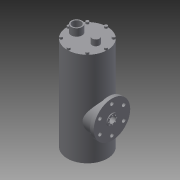
# Autodesk Inventor part: x-ray tube
Saved by Autodesk Inventor 2015 (Build 190159000, 159)
## iProperties
Created: 2014-11-30
Part Number: x-ray tube
Material: Generic
Document SubType Name: Modeling
Designer: Andrew
Density: 1 g/cm^3
Appearance: Default
Author: Andrew
Autodesk Inventor part; units mm, degrees
ref_plane "YZ Plane" through (0, 0, 0) normal (1, 0, 0) x (0, 1, 0)
ref_plane "XZ Plane" through (0, 0, 0) normal (0, 1, 0) x (-1, 0, 0)
ref_plane "XY Plane" through (0, 0, 0) normal (0, 0, 1) x (1, 0, 0)
sketch "Sketch1" plane through (0, 0, 0) normal (0, 1, 0) x (-1, 0, 0)
  circle A0 centre (0, 0) radius 34.925
  dimension "d0" = 69.85
  constraints: 1 centre point, 1 coincident
  measures "d0" diameter of A0
extrude "Extrusion1" add sketch "Sketch1" along normal blind 163.576
sketch "Sketch2" plane through (0, 0, 0) normal (1, 0, 0) x (0, 1, 0)
  circle A0 centre (62.738, 0) radius 28.575
  line L0 (0, 34.925) -> (0, -34.925) projected
  line L1 (163.576, -34.925) -> (163.576, 34.925) projected
  point P0 (0, 0)
  dimension "d3" = 100.838
  dimension "d4" = 57.15
  constraints: 1 centre point
  measures "d3" distance from line of A0.centre L1
  measures "d4" diameter of A0
extrude "Extrusion2" add sketch "Sketch2" along normal blind 36.449
sketch "Sketch3" plane through (36.449, 62.738, 0) normal (1, 0, 0) x (0, 0, -1)
  circle A0 centre (0, 0) radius 31.75
  point P0 (0, -62.738)
  dimension "d7" = 63.5
  constraints: 1 centre point
  measures "d7" diameter of A0
extrude "Extrusion3" add sketch "Sketch3" along normal blind 6.35
sketch "Sketch4" plane through (36.449, 62.738, 0) normal (-1, 0, 0) x (0, 0, 1)
  circle A0 centre (0, 0) radius 29.21
  point P0 (0, -62.738)
  dimension "d10" = 58.42
  constraints: 1 centre point
  measures "d10" diameter of A0
extrude "Extrusion4" add sketch "Sketch4" along normal blind 1.4859
sketch "Sketch5" plane through (42.799, 62.738, 0) normal (1, 0, 0) x (0, 0, -1)
  circle A0 centre (0, 0) radius 31.75 construction
  circle A1 centre (0, 0) radius 23.8125 construction
  circle A2 centre (0, 23.8125) radius 3.175
  line L0 (0, -95.4532) -> (0, 133.5532) construction
  circle A3 centre (-20.6222, 11.9063) radius 3.175
  circle A4 centre (-20.6222, -11.9062) radius 3.175
  circle A5 centre (0, -23.8125) radius 3.175
  circle A6 centre (20.6222, -11.9063) radius 3.175
  circle A7 centre (20.6222, 11.9062) radius 3.175
  circle A8 centre (0, 0) radius 5.715
  circle A9 centre (0, 0) radius 31.75 projected
  circle A10 centre (0, 0) radius 9.525
  circle A11 centre (0, 6.985) radius 0.9525
  circle A12 centre (-4.9391, 4.9391) radius 0.9525
  circle A13 centre (-6.985, 0) radius 0.9525
  circle A14 centre (-4.9391, -4.9391) radius 0.9525
  circle A15 centre (0, -6.985) radius 0.9525
  circle A16 centre (4.9391, -4.9391) radius 0.9525
  circle A17 centre (6.985, 0) radius 0.9525
  circle A18 centre (4.9391, 4.9391) radius 0.9525
  point P0 (0, -62.738)
  dimension "d13" = 47.625
  dimension "d14" = 6.35
  dimension "d17" = 360
  dimension "d19" = 11.43
  dimension "d20" = 19.05
  dimension "d21" = 1.905
  dimension "d22" = 6.985
  dimension "d25" = 360
  constraints: 16 centre point, 3 coincident, 2 point on line, 1 vertical alignment, 32 other
  measures "d14" diameter of A2
  measures "d19" diameter of A8
  measures "d20" diameter of A10
  measures "d21" diameter of A11
  measures "d22" distance of A0.centre A11.centre
extrude "Extrusion5" cut sketch "Sketch5" against normal blind 5.715 contours A2 | A3 | A4 | A5 | A6 | A7
extrude "Extrusion6" cut sketch "Sketch5" against normal blind 5.715 contours A11 | A12 | A13 | A14 | A15 | A16 | A17 | A18
extrude "Extrusion7" cut sketch "Sketch5" against normal blind 50.8 contours A8
extrude "Extrusion8" add sketch "Sketch5" along normal blind 1.27 contours A10
sketch "Sketch6" plane through (0, 163.576, 0) normal (0, 1, 0) x (1, 0, 0)
  circle A0 centre (0, 0) radius 34.925 projected
  circle A1 centre (14.6864, 0) radius 6.35
  circle A2 centre (-18.669, 0) radius 9.525
  circle A3 centre (0, -32.385) radius 2.54
  line L0 (0, 48.895) -> (0, -48.895) projected
  line L1 (59.8678, 0) -> (-50.7238, 0) projected
  circle A4 centre (0, 0) radius 29.845
  circle A5 centre (22.8997, -22.8997) radius 2.54
  circle A6 centre (32.385, 0) radius 2.54
  circle A7 centre (22.8997, 22.8997) radius 2.54
  circle A8 centre (0, 32.385) radius 2.54
  circle A9 centre (-22.8997, 22.8997) radius 2.54
  circle A10 centre (-32.385, 0) radius 2.54
  circle A11 centre (-22.8997, -22.8997) radius 2.54
  line L2 (-34.925, -31.1615) -> (-34.925, 23.8469) construction
  circle A12 centre (-18.669, 0) radius 7.62
  dimension "d35" = 5.08
  dimension "d38" = 360
  dimension "d40" = 16.256
  dimension "d41" = 12.7
  dimension "d42" = 19.05
  dimension "d43" = 15.24
  constraints: 12 centre point, 3 point on line, 3 tangent, 2 end point, 1 coincident, 1 parallel, 1 vertical, 17 other
  measures "d35" diameter of A3
  measures "d40" distance from line of L2 A2.centre
  measures "d41" diameter of A1
  measures "d42" diameter of A2
  measures "d43" diameter of A12
extrude "Extrusion9" add sketch "Sketch6" along normal blind 3.175 contours A6 L1 | L1 A6 | A7 | A5 | A8 L0 | L0 A8 | L0 A3 | A3 L0 | A9 | A11 | A10 L1 | L1 A10
extrude "Extrusion10" cut sketch "Sketch6" against normal blind 50.8 contours A12 L1 | L1 A12
extrude "Extrusion11" add sketch "Sketch6" along normal blind 12.7 contours L1 A12 A2 | A2 L1 A12
extrude "Extrusion12" add sketch "Sketch6" along normal blind 10.16 contours L1 A1 | A1 L1
ref_plane "Work Plane1" through (-22.8997, 81.788, 22.8997) normal (0, 1, 0) x (1, 0, 0)
body "Solid1"
